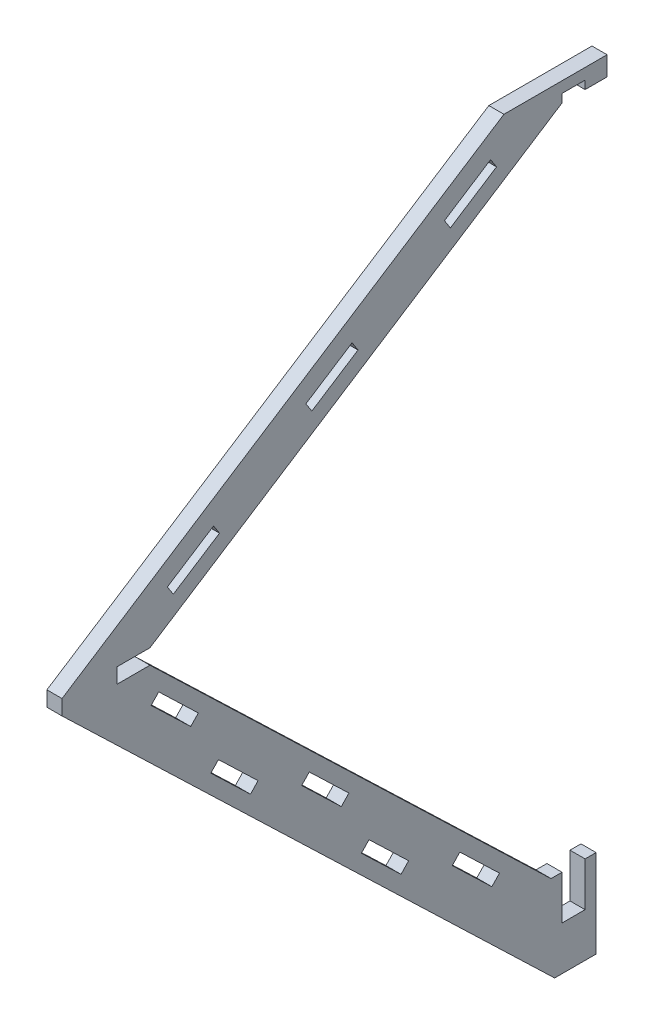
# Autodesk Inventor part: TrayPanelK
Saved by Autodesk Inventor 2017 (Build 210142000, 142)
## iProperties
Created: 2019-06-27
Part Number: TrayPanelK
Material: Generic
Document SubType Name: Modeling
Designer: DDeGo
Density: 1 g/cm^3
Appearance: Default
Author: DDeGo
Autodesk Inventor part; units mm, degrees
ref_plane "YZ Plane" through (0, 0, 0) normal (1, 0, 0) x (0, 1, 0)
ref_plane "XZ Plane" through (0, 0, 0) normal (0, 1, 0) x (-1, 0, 0)
ref_plane "XY Plane" through (0, 0, 0) normal (0, 0, 1) x (1, 0, 0)
sketch "Sketch1" plane through (0, 0, 0) normal (1, 0, 0) x (0, 1, 0)
  point P0 (0, 0)
sketch "Sketch2" plane through (0, 0, 0) normal (1, 0, 0) x (0, 1, 0)
  line L0 (0, 0) -> (0, 7.544)
  line L1 (0, 7.544) -> (86.125, 97.2)
  line L2 (86.125, 81.2) -> (16, 8.2)
  line L3 (16, 8.2) -> (16, 6.2)
  line L4 (16, 6.2) -> (8, 6.2)
  line L5 (8, 6.2) -> (8, 2)
  line L6 (8, 2) -> (16, 2)
  line L7 (16, 2) -> (16, 0)
  line L8 (16, 0) -> (0, 0)
  line L9 (88.875, 81.2) -> (137.25, 6.2)
  line L10 (137.25, 6.2) -> (138.75, 6.2)
  line L11 (138.75, 6.2) -> (138.75, 2)
  line L12 (138.75, 2) -> (137.25, 2)
  line L13 (137.25, 2) -> (137.25, -2)
  line L14 (137.25, -2) -> (140.75, -2)
  line L15 (140.75, -2) -> (140.75, 16.7736)
  line L16 (140.75, 16.7736) -> (88.875, 97.2)
  line L17 (88.875, 97.2) -> (86.125, 97.2)
  line L18 (86.125, 81.2) -> (86.125, 87.2)
  line L19 (86.125, 87.2) -> (88.875, 87.2)
  line L20 (88.875, 87.2) -> (88.875, 81.2)
  line L21 (86.125, 81.2) -> (88.875, 81.2) construction
  line L22 (137.25, 6.2) -> (137.25, 2) construction
  line L23 (86.125, 87.2) -> (86.125, 97.2) construction
  line L24 (88.875, 87.2) -> (88.875, 97.2) construction
  line L25 (137.25, 2) -> (16, 2) construction
  line L26 (16, 6.2) -> (137.25, 6.2) construction
  dimension "d0" = 4.2
  dimension "d1" = 8
  dimension "d2" = 8
  dimension "d3" = 2
  dimension "d4" = 2
  dimension "d37" = 2.75
  dimension "d38" = 75
  dimension "d39" = 86.125
  dimension "d40" = 6
  dimension "d42" = 1.5
  dimension "d43" = 2
  dimension "d44" = 4
  dimension "d45" = 10
  dimension "d47" = 138.75
  constraints: 54 end point, 10 perpendicular, 5 vertical, 4 horizontal, 4 parallel, 2 point on line
  measures "d0" distance between parallel lines of L4 L6
  measures "d1" distance between parallel lines of L3 L5
  measures "d2" distance between parallel lines of L0 L5
  measures "d3" distance of L6.end L7.end
  measures "d4" distance of L2.end L3.end
  measures "d37" distance between parallel lines of L20 L18
  measures "d38" distance from line of L2.start L4
  measures "d39" distance from line of L0 L2.start
  measures "d40" distance of L19.end L9.start
  measures "d42" distance between parallel lines of L13 L11
  measures "d43" distance between parallel lines of L15 L11
  measures "d44" distance between parallel lines of L14 L12
  measures "d45" distance between parallel lines of L17 L19
  measures "d47" distance between parallel lines of L0 L11
extrude "Extrusion1" add sketch "Sketch2" along normal blind 2.75
sketch "Sketch3" plane through (2.75, 0, 0) normal (1, 0, 0) x (0, 0, -1)
  line L0 (-79.6037, 81.125) -> (-72.3921, 74.1974)
  line L1 (-72.3921, 74.1974) -> (-73.7776, 72.755)
  line L2 (-73.7776, 72.755) -> (-80.9893, 79.6827)
  line L3 (-80.9893, 79.6827) -> (-79.6037, 81.125)
  line L4 (-8.2, 16) -> (-81.2, 86.125) projected
  line L5 (-52.1995, 54.8) -> (-44.9878, 47.8724)
  line L6 (-44.9878, 47.8724) -> (-46.3733, 46.43)
  line L7 (-46.3733, 46.43) -> (-53.585, 53.3577)
  line L8 (-53.585, 53.3577) -> (-52.1995, 54.8)
  line L9 (-24.7952, 28.475) -> (-17.5835, 21.5474)
  line L10 (-17.5835, 21.5474) -> (-18.9691, 20.105)
  line L11 (-18.9691, 20.105) -> (-26.1807, 27.0327)
  line L12 (-26.1807, 27.0327) -> (-24.7952, 28.475)
  line L13 (-70.1165, 63.5748) -> (-62.9049, 56.6471)
  line L14 (-62.9049, 56.6471) -> (-61.5193, 58.0895)
  line L15 (-61.5193, 58.0895) -> (-68.731, 65.0171)
  line L16 (-68.731, 65.0171) -> (-70.1165, 63.5748)
  line L17 (-7.544, 0) -> (-97.2, 86.125) projected
  line L18 (-68.731, 65.0171) -> (-73.7776, 72.755) construction
  line L19 (-61.5193, 58.0895) -> (-53.585, 53.3577) construction
  line L20 (-41.3267, 38.6921) -> (-42.7122, 37.2498)
  line L21 (-34.1151, 31.7645) -> (-41.3267, 38.6921)
  line L22 (-42.7122, 37.2498) -> (-35.5006, 30.3221)
  line L23 (-35.5006, 30.3221) -> (-34.1151, 31.7645)
  line L24 (-78.0276, 96.871) -> (-69.6241, 102.2913)
  line L25 (-69.6241, 102.2913) -> (-68.54, 100.6106)
  line L26 (-68.54, 100.6106) -> (-76.9436, 95.1903)
  line L27 (-76.9436, 95.1903) -> (-78.0276, 96.871)
  line L28 (-78.0276, 96.871) -> (-68.54, 100.6106) construction
  line L29 (-69.6241, 102.2913) -> (-76.9436, 95.1903) construction
  line L30 (-81.2, 88.875) -> (-6.2, 137.25) projected
  line L31 (-51.7328, 111.4512) -> (-52.8169, 113.1319)
  line L32 (-43.3292, 116.8715) -> (-51.7328, 111.4512)
  line L33 (-52.8169, 113.1319) -> (-43.3292, 116.8715) construction
  line L34 (-44.4133, 118.5523) -> (-43.3292, 116.8715)
  line L35 (-44.4133, 118.5523) -> (-51.7328, 111.4512) construction
  line L36 (-52.8169, 113.1319) -> (-44.4133, 118.5523)
  line L37 (-26.5221, 127.7122) -> (-27.6061, 129.3929)
  line L38 (-18.1185, 133.1325) -> (-26.5221, 127.7122)
  line L39 (-27.6061, 129.3929) -> (-18.1185, 133.1325) construction
  line L40 (-19.2026, 134.8132) -> (-18.1185, 133.1325)
  line L41 (-19.2026, 134.8132) -> (-26.5221, 127.7122) construction
  line L42 (-27.6061, 129.3929) -> (-19.2026, 134.8132)
  point P0 (0, 0)
  point P1 (-73.2838, 98.7408)
  point P2 (-48.0731, 115.0017)
  point P3 (-22.8623, 131.2627)
  dimension "d13" = 10
  dimension "d14" = 2
  dimension "d15" = 2.5
  dimension "d16" = 5
  dimension "d19" = 38
  dimension "d24" = 2.5
  dimension "d25" = 10
  dimension "d26" = 2
  dimension "d29" = 38
  dimension "d48" = 2
  dimension "d49" = 3
  dimension "d50" = 10
  dimension "d51" = 7
  dimension "d54" = 30
  constraints: 80 end point, 8 parallel, 6 midpoint, 3 perpendicular, 1 equal length, 49 other
  measures "d13" distance between parallel lines of L1 L3
  measures "d14" distance between parallel lines of L0 L2
  measures "d15" distance between parallel lines of L4 L0
  measures "d16" vertical distance of L4.end L0.start
  measures "d19" distance of L0.start L5.start
  measures "d24" distance between parallel lines of L17 L13
  measures "d25" distance between parallel lines of L14 L16
  measures "d26" distance between parallel lines of L15 L13
  measures "d29" distance of L15.end L20.start
  measures "d48" distance between parallel lines of L26 L24
  measures "d49" distance between parallel lines of L30 L26
  measures "d50" distance between parallel lines of L25 L27
  measures "d51" distance from line of L30.start L27
  measures "d54" distance of L26.end L31.start
extrude "Extrusion2" cut sketch "Sketch3" against normal through all
equation "\"d24\" = d15"
equation "\"d25\" = d13"
equation "\"d26\" = d14"
equation "\"d29\" = d19"
body "Solid1"
